Autodesk Inventor part; units mm, degrees
(part 2 of 2)
extrude "Extrusion91" [suppressed]
feature "Trennen15" [suppressed]
sketch "Skizze126" plane through (115.8, 0.0934, -17.5) normal (-1, 0, 0) x (0, 0, 1)
  circle A0 centre (0, 0) radius 19.4937
  point P0 (17.5, -0.0934)
  constraints: 1 centre point
extrude "Extrusion92" [suppressed]
sketch "Skizze128" plane through (115.8, 0.0934, -17.5) normal (-1, 0, 0) x (0, 0, 1)
  point P0 (17.5, -0.0934)
ref_plane "Arbeitsebene68" through (127.8, 0, -17.5) normal (1, 0, 0) x (0, 0, -1)
sketch "Skizze111" plane through (127.8, 0, -17.5) normal (1, 0, 0) x (0, 0, -1)
  circle A0 centre (0, 0) radius 13.5
  dimension "d661" = 27
  constraints: 1 centre point
  measures "d661" diameter of A0
sketch "Skizze129" plane through (106.3, 0.0934, -17.5) normal (-1, 0, 0) x (0, 0, 1)
  circle A0 centre (0, 0) radius 11.05 projected
  circle A1 centre (0, 0) radius 15 projected
  point P0 (17.5, -0.0934)
sketch "Skizze130" plane through (106.3, 0.0934, -17.5) normal (-1, 0, 0) x (0, 0, 1)
  circle A0 centre (-0.1, -0.0934) radius 14
  line L0 (-0.1, -0.0934) -> (-0.1, 2.1066) projected
  circle A1 centre (-0.1, -0.0934) radius 11.15
  circle A2 centre (-0.1, -0.0934) radius 14
  point P0 (17.5, -0.0934)
  dimension "d712" = 22.3
  dimension "d776" = 28
  constraints: 3 centre point, 2 coincident, 1 concentric
  measures "d712" diameter of A1
  measures "d776" diameter of A0
extrude "Extrusion94" [suppressed]
sketch "Skizze132" plane through (109.8, 0.0934, -17.5) normal (1, 0, 0) x (0, -0.7308407, 0.6825481)
  circle A0 centre (0, 0) radius 11.05 projected
  circle A1 centre (0, 0) radius 10.5
  circle A2 centre (0, -0.1488) radius 12.5521
  point P0 (12.0128, -12.726)
  dimension "d723" = 21
  constraints: 2 centre point, 1 coincident
  measures "d723" diameter of A1
extrude "Extrusion95" [suppressed]
sketch "Skizze131" plane through (109.8, 0.0934, -17.5) normal (1, 0, 0) x (0, -0.7045769, -0.7096277)
  arc A0 (-14, 0) -> (14, 0) centre (0, 0) ccw
  line L0 (-14, 0) -> (14, 0)
  point P0 (-12.3527, -12.3964)
  constraints: 2 end point, 2 point on circle, 1 centre point, 1 coincident, 1 horizontal
revolve "Dämpfer" add sketch "Skizze131" angle 180 about axis through (109.8, 9.9575, -7.5652) along (0, 0.7045769, 0.7096277) separate body
loft "Erhebung16" cut profiles "Skizze111", "Skizze82" bodies 6 contours all / A0
fillet "Rundung29" radius 2.5 1 edges at (119.0997, 0.0686, -7.035)
feature "Trennen16" [suppressed]
sketch "Skizze141" plane through (106.3, 0.0934, -17.5) normal (-1, 0, 0) x (0, 0, 1)
  circle A0 centre (0, 0) radius 13.1
  circle A1 centre (0, 0) radius 15.1
  circle A2 centre (0, 0) radius 17.1
  point P0 (17.5, -0.0934)
  dimension "d788" = 30.2
  dimension "d789" = 2
  dimension "d790" = 2
  constraints: 3 centre point, 2 coincident
  measures "d788" diameter of A1
  measures "d789" radial gap between concentric circles of A2 A1
  measures "d790" radial gap between concentric circles of A1 A0
extrude "DämperFormHalter" [suppressed]
extrude "Extrusion102" [suppressed]
chamfer "Fase10" [suppressed]
sketch "Skizze142" plane through (115.8, 0.0454, -17.5) normal (1, 0, 0) x (0, 0, -1)
  line L0 (6.1, -0.0454) -> (-5.9, -0.0454) projected
  circle A0 centre (0.1, -0.0454) radius 10.4477
  circle A1 centre (0, 0) radius 9.3378 projected
  point P0 (-17.5, -0.0454)
  dimension "d795" = 1
  constraints: 1 centre point
extrude "Extrusion103" [suppressed]
fillet "Rundung40" [suppressed]
